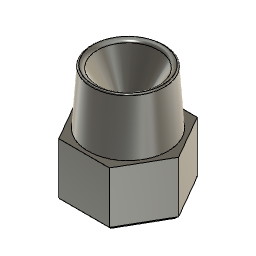
TubeNut285 (Autodesk Fusion 360 design; units mm, degrees)
Autodesk Fusion 360 part; units mm, degrees
sketch "Sketch1" plane through (0, 0, 0) normal (0, 1, 0) x (1, 0, 0)
  circle A0 centre (0, 0) radius 8
  circle A1 centre (0, 0) radius 4
  circle A2 centre (0, 0) radius 1.875
  line L0 (4.6188, -8) -> (9.2376, 0)
  line L1 (9.2376, 0) -> (4.6188, 8)
  line L2 (4.6188, 8) -> (-4.6188, 8)
  line L3 (-4.6188, 8) -> (-9.2376, 0)
  line L4 (-9.2376, 0) -> (-4.6188, -8)
  line L5 (-4.6188, -8) -> (4.6188, -8)
  dimension "d1" = 16
  dimension "d4" = 8
  dimension "d7" = 3.75
  constraint coincident A0.centre A1.centre
  constraint concentric A0 A1
  constraint horizontal L5
  constraint tangent A0 L5
  measures "d1" diameter of A0
  measures "d4" diameter of A1
  measures "d7" diameter of A2
extrude "Extrude1" add sketch "Sketch1" along normal blind 20 draft -4 contours A0 | A1 | A2
extrude "Extrude4" add sketch "Sketch1" along normal blind 10 contours A0 | A0 L0 L1 | A0 L1 L2 | A0 L0 L5 | A0 L2 L3 | A0 L4 L5 | A0 L3 L4 | A1 | A2
extrude "Extrude3" cut sketch "Sketch1" along normal through all contours A2
chamfer "Chamfer1" distance 4 angle 60 1 edges at (-1.7481, 20, -0.678) measured on face at (5.0014, 20, -0.328)
fillet "Fillet1" radius 1 1 edges at (-5.4774, 20, 2.1245)
fillet "Fillet2" radius 3 1 edges at (-1.7481, 13.0718, -0.678)
fillet "Fillet3" radius 0.25 1 edges at (-6.1547, 20, -2.3872)
sketch "Sketch2" plane through (0, 0, 0) normal (0, 0, 1) x (1, 0, 0)
  line L0 (-36, 0) -> (36, 0) construction
  line L1 (0, 34.3715) -> (0, -34.3715) construction
  line L2 (0, 0) -> (-4.5, 0)
  line L3 (-4.5, 8) -> (0, 12.5)
  line L4 (-4.5, 8) -> (-4.5, 0)
  line L5 (0, 12.5) -> (0, 0)
  line L6 (-4.5, 0) -> (0, 0)
  dimension "d24" = 4.5
  dimension "d25" = 45
  dimension "d27" = 8
  constraint vertical L1
  constraint horizontal L0
  constraint midpoint L2.start L1
  constraint midpoint L2.start L0
  constraint coincident L2.start L5.end
  constraint coincident L0 L2.end
  constraint perpendicular L1 L2
  constraint coincident L1 L3.end
  constraint perpendicular L0 L4
  measures "d24" distance of L1 L4
  measures "d25" angle of L1 L3
  measures "d27" distance of L2.end L3.start
revolve "Revolve1" cut sketch "Sketch2" angle 360 about axis through (0, 34.3715, 0) along (0, -1, 0)
fillet "Fillet4" radius 1 1 edges at (-1.7481, 10.625, -0.678)
chamfer "Chamfer4" distance 0.6 angle 45 7 edges at (0, 0, 8) (-6.9282, 0, 4) (-6.9282, 0, -4) (6.9282, 0, 4) (6.9282, 0, -4) (0, 0, -8) (4.1955, 0, -1.6273)
move_body "Move1" bodies 1 to x (1, 0, 0) y (0, 0, 1) z (0, -1, 0) at (0, 5, -5)
equation "d24 = BSP / 2"
equation "BSP = 9 mm"
